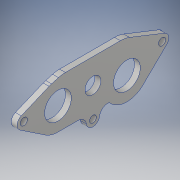
# Autodesk Inventor part: Gearbox Plate 1
Saved by Autodesk Inventor 2019.4 (Build 234330000, 330)
## iProperties
Created: 2019-12-11
Part Number: Gearbox Plate 1
Material: Aluminum 6061
Document SubType Name: Modeling
Designer: admin
Density: 2.7 g/cm^3
Appearance: Aluminum - Flat
Mass: 130.89 g
Surface Area: 192.187 cm^2
Volume: 48.4777 cm^3
Author: admin
Autodesk Inventor part; units mm, degrees
ref_plane "YZ Plane" through (0, 0, 0) normal (1, 0, 0) x (0, 1, 0)
ref_plane "XZ Plane" through (0, 0, 0) normal (0, 1, 0) x (-1, 0, 0)
ref_plane "XY Plane" through (0, 0, 0) normal (0, 0, 1) x (1, 0, 0)
sketch "Sketch6" plane through (0, 0, 0) normal (1, 0, 0) x (0, 1, 0)
  circle A0 centre (0, 0) radius 9.5
  circle A1 centre (-10, -40.7922) radius 16
  circle A2 centre (0, 42) radius 16
  line L0 (0, 0) -> (0, -14.5947) construction
  line L1 (0, 0) -> (0, -33.02)
  line L2 (0, 0) -> (33.02, 0) construction
  circle A3 centre (0, -33.02) radius 30
  line L3 (0, 0) -> (0, 33.02)
  line L4 (0, 0) -> (33.02, 0) construction
  circle A4 centre (0, 33.02) radius 30
  line L5 (0, 0) -> (-10, -40.7922)
  line L6 (0, 0) -> (0, 42)
  circle A5 centre (0, 42) radius 27.5
  circle A6 centre (-10, -40.7922) radius 27.5
  line L7 (30, 33.02) -> (30, -33.02)
  line L8 (-27.5, 42) -> (-27.5, -19.579)
  line L9 (26.4128, 49.6559) -> (28.814, 41.3719)
  line L10 (2.2577, -65.4092) -> (13.3721, -59.8749)
  dimension "d45" = 19
  dimension "d46" = 32
  dimension "d47" = 32
  dimension "d50" = 0
  dimension "d51" = 10
  dimension "d52" = 33.02
  dimension "d53" = 90
  dimension "d54" = 60
  dimension "d55" = 33.02
  dimension "d56" = 90
  dimension "d57" = 60
  dimension "d58" = 42
  dimension "d59" = 42
  dimension "d60" = 55
  dimension "d61" = 55
  constraints: 22 end point, 8 point on circle, 7 centre point, 7 coincident, 7 tangent, 2 collinear, 2 horizontal, 2 perpendicular, 2 vertical
  measures "d45" diameter of A0
  measures "d46" diameter of A1
  measures "d47" diameter of A2
  measures "d50" distance from line of L0 A2.centre
  measures "d51" distance from line of A1.centre L0
  measures "d52" distance of L0.start L1.end
  measures "d53" angle of L1 L2
  measures "d54" diameter of A3
  measures "d55" distance of L0.start L3.end
  measures "d56" angle of L4 L3
  measures "d57" diameter of A4
  measures "d58" distance of L0.start L5.end
  measures "d59" distance of L0.start L6.end
  measures "d60" diameter of A5
  measures "d61" diameter of A6
extrude "Extrusion6" add sketch "Sketch6" along normal blind 7 contours A0 A3 L1 L3 A4 | A0 A4 L7 A3 | A4 L3 A0 | A0 L3 A5 A4 | A3 A6 L1 A0 | A0 L1 A3 | L3 A4 A0 | A0 A4 L8 A5 L3 | L3 L5 A3 A0 A4 | L1 A6 L5 A0 | A0 L5 A3 L1 | A3 L5 L1 | A0 A3 A6 L8 A4 | A5 A4 | A4 A5 L9 | L5 A6 A3 A0 | A0 A3 L5 | A6 A3 L5 A1 L1 | L1 A1 L5 A6 | L10 A6 A3 | A4 A5 | A1 | A6 A3 | A2
sketch "Sketch7" plane through (7, 0, 0) normal (1, 0, 0) x (0, 0, -1)
  circle A0 centre (0, 0) radius 9.5
  circle A1 centre (40.7922, -10) radius 16
  circle A2 centre (-42, 0) radius 16
  line L0 (0, 0) -> (40.7922, -10) construction
  line L1 (0, 0) -> (-42, 0) construction
  dimension "d64" = 19
  dimension "d65" = 32
  dimension "d66" = 32
  dimension "d67" = 0
  dimension "d70" = 42
  dimension "d71" = 42
  dimension "d102" = 10
  constraints: 5 end point, 3 centre point, 2 coincident
  measures "d64" diameter of A0
  measures "d65" diameter of A1
  measures "d66" diameter of A2
  measures "d67" vertical distance of L0.start A2.centre
  measures "d70" distance of L0.end L0.start
  measures "d71" distance of L0.start L1.end
  measures "d102" vertical distance of L0.start L0.end
extrude "Extrusion7" cut sketch "Sketch7" against normal blind 10
sketch "Sketch11" plane through (7, 0, 0) normal (1, 0, 0) x (0, 0, -1)
  circle A0 centre (0, -35) radius 4
  circle A1 centre (0, -35) radius 8
  arc A2 (-49.6559, 26.4128) -> (-42, -27.5) centre (-42, 0) ccw projected
  line L0 (33.02, 30) -> (-33.02, 30) projected
  arc A3 (19.579, -27.5) -> (65.4092, 2.2577) centre (40.7922, -10) ccw projected
  circle A4 centre (-83.02, 4) radius 4.25
  circle A5 centre (-83.02, 4) radius 8
  line L1 (-86.1032, 11.382) -> (-52.5984, 25.3756)
  line L2 (-87.4712, -2.6473) -> (-57.3011, -22.8501)
  line L3 (-57.3011, -22.8501) -> (-64.274, 6.2236)
  line L4 (-64.274, 6.2236) -> (-52.5984, 25.3756)
  line L5 (0, 0) -> (0, -10)
  line L6 (0, 0) -> (10, 0) construction
  circle A6 centre (83.02, 4) radius 4.25
  circle A7 centre (83.02, 4) radius 8
  line L7 (88.2989, -2.0111) -> (60.0176, -29.663)
  line L8 (86.7797, 11.0615) -> (44.0182, 27.9113)
  arc A8 (59.8749, 13.3721) -> (33.02, 30) centre (33.02, 0) ccw projected
  line L9 (60.0176, -29.663) -> (63.5624, -5)
  line L10 (63.5624, -5) -> (44.0182, 27.9113)
  dimension "d94" = 16
  dimension "d103" = 8.5
  dimension "d104" = 16
  dimension "d105" = 83.02
  dimension "d106" = 4
  dimension "d107" = 10
  dimension "d108" = 90
  constraints: 20 end point, 8 point on circle, 6 centre point, 6 tangent, 3 coincident, 2 symmetric about line, 1 horizontal, 1 perpendicular, 1 vertical, 4 other
  measures "d94" diameter of A1
  measures "d103" diameter of A4
  measures "d104" diameter of A5
  measures "d105" horizontal distance of L5.start A5.centre
  measures "d106" vertical distance of L5.start A5.centre
  measures "d107" distance of L5.start L5.end
  measures "d108" angle of L5 L6
extrude "Extrusion10" add sketch "Sketch11" against normal blind 7 contours A1 | L4 L3 A2 | A2 L2 A5 L1 | A5 | A4 | A6 | A7 L8 | L7 L9 L10 L8 A7 picked at (83.9305, 10.6486)
fillet "Fillet4" radius 10 2 edges at (3.5, -27.5, -2.7839) (3.5, -27.5, 2.7839)
sketch "Sketch12" plane through (7, 0, 0) normal (1, 0, 0) x (0, 0, -1)
  circle A0 centre (-83.02, 20) radius 4.25
  circle A1 centre (83.02, 20) radius 4.25
  arc A2 (91.2252, 14.2838) -> (83.02, 30) centre (83.02, 20) ccw projected
  arc A3 (-83.02, 30) -> (-90.5143, 13.3792) centre (-83.02, 20) ccw projected
  point P0 (0, 0)
  dimension "d98" = 8.5
  dimension "d99" = 8.5
  constraints: 2 centre point, 2 concentric
  measures "d98" diameter of A0
  measures "d99" diameter of A1
extrude "Extrusion11" cut sketch "Sketch12" against normal blind 10
sketch "Sketch13" plane through (7, 0, 0) normal (1, 0, 0) x (0, 0, -1)
  circle A0 centre (-83.02, 4) radius 4.25
  circle A1 centre (83.02, 4) radius 4.25
  arc A2 (88.2989, -2.0111) -> (86.7797, 11.0615) centre (83.02, 4) ccw projected
  arc A3 (-86.1032, 11.382) -> (-87.4712, -2.6473) centre (-83.02, 4) ccw projected
  point P0 (0, 0)
  dimension "d109" = 8.5
  dimension "d110" = 8.5
  constraints: 2 centre point, 2 concentric
  measures "d109" diameter of A0
  measures "d110" diameter of A1
extrude "Extrusion12" cut sketch "Sketch13" against normal blind 10
body "Solid2"
